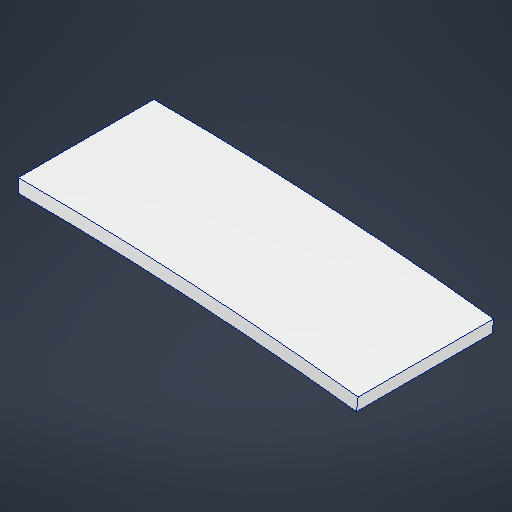
# Autodesk Inventor part: Doubler Plate, Bolted and Welded
Saved by Autodesk Inventor 2026 (Build 300175000, 175)
## iProperties
Created: 2025-11-03
Part Number: Doubler Plate, Bolted and Welded
Material: Aluminum 6061
Document SubType Name: Modeling
Designer: Brandon Portillo
Density: 2.7 g/cm^3
Appearance: Aluminum - Flat
Author: Brandon Portillo
Autodesk Inventor part; units mm, degrees
ref_plane "YZ Plane" through (0, 0, 0) normal (1, 0, 0) x (0, 1, 0)
ref_plane "XZ Plane" through (0, 0, 0) normal (0, 1, 0) x (-1, 0, 0)
ref_plane "XY Plane" through (0, 0, 0) normal (0, 0, 1) x (1, 0, 0)
sketch "Sketch1" plane through (0, 0, 0) normal (0, 0, 1) x (1, 0, 0)
  arc A0 (250.7437, 2105.1194) -> (0, 2120) centre (0, 0) ccw
  arc A1 (249.5609, 2095.1896) -> (0, 2110) centre (0, 0) ccw
  line L0 (0, 2110) -> (0, 2120)
  arc A2 (249.5609, 2095.1896) -> (0, 2110) centre (0, 0) ccw
  line L1 (249.5609, 2095.1896) -> (250.7437, 2105.1194)
  arc A3 (250.7437, 2105.1194) -> (0, 2120) centre (0, 0) ccw
  dimension "d1" = 4240
  dimension "d2" = 4220
  dimension "d4" = 250
  dimension "d5" = 10
  constraints: 8 point on circle, 4 centre point, 4 end point, 2 coincident, 1 vertical
  measures "d1" diameter of A0
  measures "d2" diameter of A1
  measures "d4" distance of L0.start L1.start
  measures "d5" distance of L1.start L1.end
extrude "Extrusion1" add sketch "Sketch1" along normal blind 100
body "Solid1"
